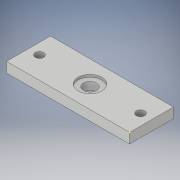
# Autodesk Inventor part: top plate
Saved by Autodesk Inventor 2018 (Build 220112000, 112)
## iProperties
Created: 2018-07-18
Part Number: top plate
Material: Generic
Document SubType Name: Modeling
Designer: BB-8
Density: 1 g/cm^3
Appearance: Default
Author: BB-8
Autodesk Inventor part; units mm, degrees
ref_plane "YZ Plane" through (0, 0, 0) normal (1, 0, 0) x (0, 1, 0)
ref_plane "XZ Plane" through (0, 0, 0) normal (0, 1, 0) x (-1, 0, 0)
ref_plane "XY Plane" through (0, 0, 0) normal (0, 0, 1) x (1, 0, 0)
sketch "Sketch2" plane through (0, 0, 0) normal (0, 1, 0) x (-1, 0, 0)
  line L0 (0, 0) -> (280, 0)
  line L1 (280, 0) -> (280, -100)
  line L2 (280, -100) -> (0, -100)
  line L3 (0, -100) -> (0, 0)
  circle A0 centre (140, -50) radius 15
  circle A1 centre (255, -50) radius 9.5
  circle A2 centre (25, -50) radius 9.5
  dimension "d0" = 280
  dimension "d1" = 100
  dimension "d2" = 30
  dimension "d3" = 19
  dimension "d4" = 19
  dimension "d5" = 115
  dimension "d6" = 115
  constraints: 8 end point, 3 centre point, 2 parallel, 1 horizontal, 1 perpendicular
  measures "d0" distance of L1.end L2.end
  measures "d1" distance of L0.end L1.end
  measures "d2" diameter of A0
  measures "d3" diameter of A1
  measures "d4" diameter of A2
  measures "d5" distance of A0.centre A2.centre
  measures "d6" distance of A1.centre A0.centre
extrude "Extrusion2" add sketch "Sketch2" along normal blind 23
sketch "Sketch4" plane through (0, 23, 0) normal (0, 1, 0) x (1, 0, 0)
  circle A0 centre (-140, 50) radius 27
  point P0 (0, 0)
  dimension "d11" = 54
  constraints: 1 centre point
  measures "d11" diameter of A0
extrude "Extrusion3" cut sketch "Sketch4" against normal blind 5
sketch "Sketch5" plane through (0, 23, 0) normal (0, 1, 0) x (1, 0, 0)
  point P0 (0, 0)
body "Solid2"
